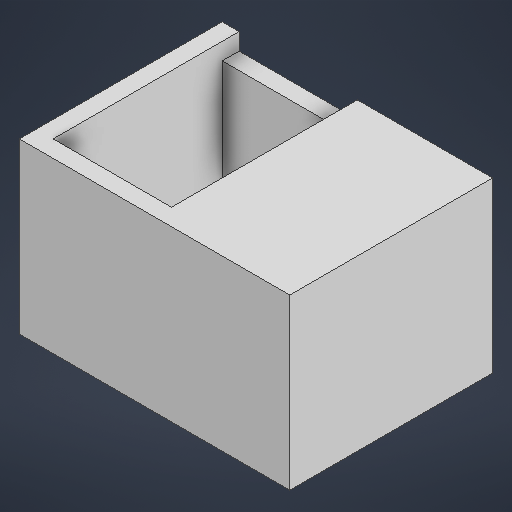
# Autodesk Inventor part: rightcollection
Saved by Autodesk Inventor 2026.2 (Build 302298000, 298)
## iProperties
Created: 2026-04-08
Part Number: rightcollection
Material: Generic
Document SubType Name: Modeling
Designer: danda
Density: 1 g/cm^3
Appearance: Default
Author: danda
Autodesk Inventor part; units mm, degrees
ref_plane "YZ Plane" through (0, 0, 0) normal (1, 0, 0) x (0, 1, 0)
ref_plane "XZ Plane" through (0, 0, 0) normal (0, 1, 0) x (-1, 0, 0)
ref_plane "XY Plane" through (0, 0, 0) normal (0, 0, 1) x (1, 0, 0)
sketch "Sketch1" plane through (0, 0, 0) normal (0, 0, 1) x (1, 0, 0)
  line L0 (23.2261, 43.4376) -> (23.2261, 3.4376)
  line L1 (23.2261, 43.4376) -> (93.2261, 43.4376)
  line L2 (93.2261, 43.4376) -> (93.2261, 3.4376)
  line L3 (93.2261, 3.4376) -> (23.2261, 3.4376)
  line L4 (23.2261, 3.4376) -> (93.2261, 13.4376)
  line L5 (58.2261, 8.4376) -> (58.2261, 3.4376)
  line L6 (98.2261, 48.4376) -> (18.2261, 48.4376)
  line L7 (18.2261, 48.4376) -> (18.2261, -1.5624)
  line L8 (18.2261, -1.5624) -> (98.2261, -1.5624)
  line L9 (98.2261, -1.5624) -> (98.2261, 48.4376)
  line L10 (23.2261, 43.4376) -> (23.2261, 48.4376)
  line L11 (93.2261, 43.4376) -> (93.2261, 48.4376)
  line L12 (58.2261, 43.4376) -> (58.2261, 48.4376)
  point P0 (0, 0)
  dimension "d0" = 40
  dimension "d1" = 70
  dimension "d2" = 10
  dimension "d4" = 5
  dimension "d5" = 5
  dimension "d16" = 35
  constraints: 26 end point, 8 perpendicular, 4 midpoint, 3 point on line, 2 vertical, 1 horizontal, 3 other
  measures "d0" distance of L0.start L0.end
  measures "d1" distance of L0.start L1.end
  measures "d2" distance of L2.end L4.end
  measures "d4" distance of L5.start L5.end
  measures "d5" distance between parallel lines of L1 L6
  measures "d16" distance between parallel lines of L11 L12
extrude "Extrusion1" add sketch "Sketch1" along normal blind 60 contours L10 L6 L12 L1 | L0 L3 L2 L11 L6 L9 L8 L7 L10
extrude "Extrusion2" add sketch "Sketch1" along normal blind 5 contours L1 L2 L4 L0
extrude "Extrusion3" add sketch "Sketch1" along normal blind 60 contours L5 L4 L2 L3
sketch "Sketch2" plane through (18.2261, -1.5624, 0) normal (-1, 0, 0) x (0, 0, 1)
  line L0 (60, 0) -> (60, 50) projected
  line L1 (60, 0) -> (60, 5)
  line L2 (5, 10) -> (60, 10) projected
  line L3 (60, 5) -> (5, 10)
  line L4 (5, 5) -> (5, 45) projected
  line L5 (5, 5) -> (5, 10)
  line L6 (5, 5) -> (60, 5)
  point P0 (0, 1.5624)
  dimension "d12" = 5
  constraints: 8 end point, 1 collinear, 1 point on line
  measures "d12" distance of L0.start L1.end
extrude "Extrusion4" add sketch "Sketch2" against normal blind 45 contours L6 L4 L3
sketch "Sketch3" plane through (0, 0, 60) normal (0, 0, 1) x (1, 0, 0)
  line L0 (18.2261, 48.4376) -> (18.2261, -1.5624) projected
  line L1 (18.2261, -1.5624) -> (98.2261, -1.5624) projected
  line L2 (18.2261, 48.4376) -> (98.2261, 48.4376)
  line L3 (98.2261, 48.4376) -> (98.2261, -1.5624)
  line L4 (98.2261, -1.5624) -> (18.2261, -1.5624)
  line L5 (18.2261, -1.5624) -> (18.2261, 48.4376)
  point P0 (0, 0)
  constraints: 8 end point, 2 parallel, 1 horizontal, 1 perpendicular
extrude "Extrusion5" add sketch "Sketch3" against normal blind 5
sketch "Sketch4" plane through (18.2261, -1.5624, 0) normal (0, -1, 0) x (1, 0, 0)
  line L0 (0, 0) -> (0, 60) projected
  line L1 (0, 60) -> (40, 60)
  line L2 (40, 60) -> (40, 25)
  line L3 (40, 25) -> (0, 25)
  line L4 (0, 25) -> (0, 60)
  line L5 (5, 55) -> (5, 5) projected
  line L6 (5, 25) -> (5, 55)
  line L7 (5, 55) -> (40, 55)
  point P0 (-18.2261, 0)
  point P1 (0, 25)
  dimension "d19" = 40
  dimension "d20" = 35
  constraints: 12 end point, 3 point on line, 2 parallel, 2 perpendicular, 1 collinear, 1 horizontal
  measures "d19" distance of L2.end L3.end
  measures "d20" distance of L1.end L2.end
extrude "Extrusion6" cut sketch "Sketch4" against normal blind 10 contours L5 L7 L2 L3
mirror "Mirror1" about plane through (0, 0, 0) normal (1, 0, 0) remove original yes
body "Solid1"
